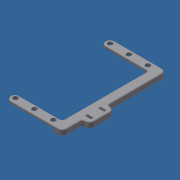
# Autodesk Inventor part: MotorServo2
Saved by Autodesk Inventor 2015 SP1 (Build 190203100, 203)
## iProperties
Created: 2015-11-11
Part Number: MotorServo2
Material: Generic
Document SubType Name: Modeling
Designer: Dale
Density: 1 g/cm^3
Appearance: Default
Author: Dale
Autodesk Inventor part; units mm, degrees
ref_plane "YZ Plane" through (0, 0, 0) normal (1, 0, 0) x (0, 1, 0)
ref_plane "XZ Plane" through (0, 0, 0) normal (0, 1, 0) x (-1, 0, 0)
ref_plane "XY Plane" through (0, 0, 0) normal (0, 0, 1) x (1, 0, 0)
sketch "Sketch1" plane through (0, 0, 0) normal (0, 0, 1) x (1, 0, 0)
  line L0 (-20, -40) -> (-20, -40)
  line L1 (-16.5, -36.5) -> (18, -36.5)
  line L2 (20, -34.5) -> (20, 34.5)
  line L3 (18, 36.5) -> (-16.5, 36.5)
  line L4 (-20, 40) -> (-20, 40)
  line L5 (-16, 44) -> (24, 44)
  line L6 (28, 40) -> (28, -4)
  line L7 (30, -6) -> (30, -6)
  line L8 (34, -10) -> (34, -23)
  line L9 (30, -27) -> (30, -27)
  line L10 (28, -29) -> (28, -40)
  line L11 (24, -44) -> (-16, -44)
  arc A0 (-20, -40) -> (-16, -44) centre (-16, -40) ccw
  arc A1 (24, -44) -> (28, -40) centre (24, -40) ccw
  arc A2 (-16, 44) -> (-20, 40) centre (-16, 40) ccw
  arc A3 (28, 40) -> (24, 44) centre (24, 40) ccw
  arc A4 (20, 34.5) -> (18, 36.5) centre (18, 34.5) ccw
  arc A5 (28, -4) -> (30, -6) centre (30, -4) ccw
  arc A6 (30, -27) -> (28, -29) centre (30, -29) ccw
  arc A7 (18, -36.5) -> (20, -34.5) centre (18, -34.5) ccw
  arc A8 (34, -10) -> (30, -6) centre (30, -10) ccw
  arc A9 (30, -27) -> (34, -23) centre (30, -23) ccw
  arc A10 (-16.5, -36.5) -> (-20, -40) centre (-16.5, -40) ccw
  arc A11 (-20, 40) -> (-16.5, 36.5) centre (-16.5, 40) ccw
  point P0 (0, 0)
  point P1 (-20, 36.5)
  point P2 (-20, 44)
  point P3 (28, -6)
  point P4 (34, -6)
  point P5 (28, -27)
  point P6 (28, -44)
  dimension "d0" = 88
  dimension "d1" = 44
  dimension "d2" = 48
  dimension "d3" = 40
  dimension "d5" = 20
  dimension "d6" = 7.5
  dimension "d7" = 7.5
  dimension "d8" = 6
  dimension "d9" = 17
  dimension "d11" = 4
  dimension "d12" = 2
  dimension "d13" = 4
  dimension "d14" = 3.5
  dimension "d53" = 21
  constraints: 24 end point, 24 point on circle, 24 tangent, 16 point on line, 12 centre point, 8 equal radius, 6 horizontal, 4 vertical
  measures "d0" distance between parallel lines of L11 L5
  measures "d1" distance from line of point (0, 0) L5
  measures "d2" distance between parallel lines of L6 L4
  measures "d3" distance between parallel lines of L2 L4
  measures "d5" distance from line of point (0, 0) L2
  measures "d6" distance between parallel lines of L11 L1
  measures "d7" distance between parallel lines of L3 L5
  measures "d8" distance of point (28, -6) point (34, -6)
  measures "d9" distance between parallel lines of L11 L9
  measures "d11" radius of A0
  measures "d12" radius of A4
  measures "d13" radius of A8
  measures "d14" radius of A10
  measures "d53" distance of L7.start L9.end
extrude "Base" add sketch "Sketch1" along normal blind 5.2
sketch "Sketch2" plane through (0, 0, 5.2) normal (0, 0, 1) x (1, 0, 0)
  circle A0 centre (-16, -40) radius 2.05
  line L0 (-16, -44) -> (24, -44) projected
  line L1 (34, -24) -> (34, -10) construction
  circle A1 centre (0, -40) radius 2.05
  circle A2 centre (16, -40) radius 2.05
  circle A3 centre (-16, 40) radius 2.05
  circle A4 centre (0, 40) radius 2.05
  circle A5 centre (16, 40) radius 2.05
  point P0 (0, 0)
  point P1 (-20, -40)
  point P2 (-20, -40)
  dimension "d17" = 4.1
  dimension "d18" = 4
  dimension "d19" = 4
  dimension "d22" = 16
  dimension "d25" = 80
  dimension "d28" = 20
  constraints: 6 centre point, 2 end point, 2 vertical, 1 coincident, 1 horizontal, 10 other
  measures "d17" diameter of A0
  measures "d18" distance from line of A0.centre L0
  measures "d19" distance of point (-20, -40) A0.centre
  measures "d22" distance of A0.centre A1.centre
  measures "d25" distance of A0.centre A3.centre
  measures "d28" distance from line of L1.start L0
extrude "Mounting Holes" cut sketch "Sketch2" against normal through all
sketch "Sketch3" plane through (0, 0, 5.2) normal (0, 0, 1) x (1, 0, 0)
  line L0 (26.5, -21) -> (31, -21)
  line L1 (31, -21) -> (31, -23)
  line L2 (31, -23) -> (26.5, -23)
  line L3 (26.5, -23) -> (26.5, -21)
  line L4 (-16, -44) -> (24, -44) projected
  line L5 (20, 34.5) -> (20, -34.5) projected
  line L6 (26.5, -10) -> (31, -10)
  line L7 (31, -10) -> (31, -12)
  line L8 (31, -12) -> (26.5, -12)
  line L9 (26.5, -12) -> (26.5, -10)
  point P0 (0, 0)
  dimension "d31" = 21
  dimension "d32" = 2
  dimension "d33" = 4.5
  dimension "d34" = 6.5
  dimension "d37" = 11
  constraints: 16 end point, 2 parallel, 1 horizontal, 1 perpendicular, 1 vertical, 8 other
  measures "d31" distance between parallel lines of L2 L4
  measures "d32" distance between parallel lines of L2 L0
  measures "d33" distance of L1.end L2.end
  measures "d34" distance between parallel lines of L3 L5
  measures "d37" distance of L0.start L6.start
extrude "Zip Tie Slot" cut sketch "Sketch3" against normal through all
sketch "Sketch4" plane through (0, 0, 0) normal (0, 0, -1) x (-1, 0, 0)
  line L0 (16, 44) -> (-24, 44) projected
  line L1 (-20, 44) -> (20, 44)
  line L2 (20, 44) -> (20, -44)
  line L3 (20, -44) -> (-20, -44)
  line L4 (-20, -44) -> (-20, 44)
  line L5 (-24, -44) -> (16, -44) projected
  line L6 (-20, -34.5) -> (-20, 34.5) projected
  arc A0 (16, 44) -> (16, 44) centre (16, 40) ccw projected
  point P0 (0, 0)
  point P1 (20, 40)
  constraints: 8 end point, 2 collinear, 2 parallel, 1 horizontal, 1 perpendicular, 1 point on line, 1 vertical, 1 other
extrude "Mount Cutout" cut sketch "Sketch4" against normal blind 3
sketch "Sketch5" plane through (0, 0, 0) normal (0, 0, -1) x (-1, 0, 0)
  line L0 (-31, -12) -> (-26.5, -12)
  line L1 (-26.5, -12) -> (-26.5, -21)
  line L2 (-26.5, -21) -> (-31, -21)
  line L3 (-31, -21) -> (-31, -12)
  line L4 (-26.5, -12) -> (-31, -12) projected
  line L5 (-31, -12) -> (-31, -10) projected
  point P0 (0, 0)
  constraints: 8 end point, 2 collinear, 2 parallel, 1 horizontal, 1 perpendicular
extrude "Zip Tie Cutout" cut sketch "Sketch5" against normal blind 2
fillet "Rounded Zip Tie Strap" radius 2 2 edges at (28.75, -21, 2) (28.75, -12, 2)
fillet "Rounded Cutout" radius 0.8 4 edges at (28.75, -10, 0) (31, -16.5, 0) (28.75, -23, 0) (26.5, -16.5, 0)
fillet "Rounded Top" radius 1 20 edges at (20, 0, 5.2) (19.4142, -35.9142, 5.2) (0.75, -36.5, 5.2) (-18.9749, -37.5251, 5.2) (-18.8284, -42.8284, 5.2) (4, -44, 5.2) (26.8284, -42.8284, 5.2) (28, -34.5, 5.2) (28.5858, -27.5858, 5.2) (32.8284, -25.8284, 5.2) (34, -16.5, 5.2) (32.8284, -7.1716, 5.2) (28.5858, -5.4142, 5.2) (28, 18, 5.2) (26.8284, 42.8284, 5.2) (4, 44, 5.2) (-18.8284, 42.8284, 5.2) (-18.9749, 37.5251, 5.2) (0.75, 36.5, 5.2) (19.4142, 35.9142, 5.2)
fillet "Rounded Bottom" radius 1 11 edges at (28, 18, 0) (26.8284, 42.8284, 0) (22, 44, 0) (28.5858, -5.4142, 0) (32.8284, -7.1716, 0) (34, -16.5, 0) (32.8284, -25.8284, 0) (28.5858, -27.5858, 0) (28, -34.5, 0) (26.8284, -42.8284, 0) (22, -44, 0)
fillet "Rounded Slots" radius 0.8 8 edges at (28.75, -10, 5.2) (31, -11, 5.2) (28.75, -12, 5.2) (26.5, -11, 5.2) (28.75, -21, 5.2) (28.75, -23, 5.2) (31, -22, 5.2) (26.5, -22, 5.2)
body "Solid1"
